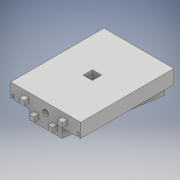
# Autodesk Inventor part: tb3_start
Saved by Autodesk Inventor 2017 (Build 210142000, 142)
## iProperties
Created: 2017-02-24
Part Number: tb3_start
Material: Generic
Document SubType Name: Modeling
Designer: PC
Density: 1 g/cm^3
Appearance: Default
Author: PC
Autodesk Inventor part; units mm, degrees
ref_plane "YZ Plane" through (0, 0, 0) normal (1, 0, 0) x (0, 1, 0)
ref_plane "XZ Plane" through (0, 0, 0) normal (0, 1, 0) x (-1, 0, 0)
ref_plane "XY Plane" through (0, 0, 0) normal (0, 0, 1) x (1, 0, 0)
sketch "Sketch5" plane through (0, 0, 0) normal (0, 1, 0) x (-1, 0, 0)
  line L0 (-37.5, -7.5) -> (37.5, -7.5)
  line L1 (37.5, -7.5) -> (37.5, 7.5)
  line L2 (37.5, 7.5) -> (-37.5, 7.5)
  line L3 (-37.5, 7.5) -> (-37.5, -7.5)
  line L4 (-37.5, -7.5) -> (37.5, 7.5) construction
  line L5 (37.5, -7.5) -> (-37.5, 7.5) construction
  point P0 (0, 0)
  dimension "d6" = 75
  dimension "d7" = 15
  constraints: 12 end point, 2 midpoint, 2 parallel, 1 horizontal, 1 perpendicular
  measures "d6" distance of L2.end L1.end
  measures "d7" distance of L1.end L0.end
extrude "Extrusion2" add sketch "Sketch5" along normal blind 100
sketch "Sketch36" plane through (0, 0, 0) normal (0, -1, 0) x (1, 0, 0)
  line L0 (-37.5, 7.5) -> (37.5, 7.5) projected
  line L1 (0, 7.5) -> (0, -2.5)
  point P0 (0, 0)
  dimension "d82" = 10
  constraints: 2 end point, 1 midpoint, 1 vertical
  measures "d82" distance of L1.start L1.end
hole "Hole1" at (0, 0, -2.5) direction (0, 1, 0) diameter 6.4 depth 10 tip angle 118
sketch "Sketch37" plane through (37.5, 0, -7.5) normal (0, 0, -1) x (-1, 0, 0)
  line L0 (37.5, 0) -> (55, 0)
  line L1 (75, 0) -> (0, 0) projected
  line L2 (70, 0) -> (70, 95)
  line L3 (0, 100) -> (75, 100) projected
  line L4 (70, 0) -> (165, 0) construction
  line L5 (70, 95) -> (5, 95)
  line L6 (0, 0) -> (0, 100) projected
  line L7 (5, 95) -> (5, 0)
  line L8 (5, 0) -> (0, 0)
  line L9 (0, 100) -> (75, 100)
  line L10 (75, 100) -> (75, 0)
  line L11 (55, 0) -> (70, 95)
  line L12 (5, 95) -> (70, 95)
  line L13 (37.5, 0) -> (20, 0)
  line L14 (20, 0) -> (5, 95)
  dimension "d90" = 17.5
  dimension "d91" = 95
  dimension "d92" = 90
  dimension "d93" = 65
  dimension "d94" = 17.5
  constraints: 24 end point, 6 perpendicular, 4 point on line, 2 horizontal, 1 collinear
  measures "d90" distance of L0.start L0.end
  measures "d91" distance of L2.start L2.end
  measures "d92" angle of L4 L2
  measures "d93" distance of L2.end L5.end
  measures "d94" distance of L0.start L13.end
extrude "Extrusion11" add sketch "Sketch37" along normal blind 10 contours L1 L14 L5 L11 L0
sketch "Sketch38" plane through (37.5, 100, -7.5) normal (0, 0, -1) x (-1, 0, 0)
  line L0 (75, -100) -> (0, -100) projected
  line L1 (1.5, -100) -> (3.5, -100)
  line L2 (3.5, -100) -> (3.5, -1.5)
  line L3 (3.5, -1.5) -> (1.5, -1.5)
  line L4 (1.5, -1.5) -> (1.5, -100)
  line L5 (1.5, -1.5) -> (73.5, -1.5)
  line L6 (73.5, -1.5) -> (73.5, -3)
  line L7 (73.5, -3) -> (1.5, -3)
  line L8 (1.5, -3) -> (1.5, -1.5)
  line L9 (55, -100) -> (75, -100) projected
  line L10 (73.5, -1.5) -> (71.5, -1.5)
  line L11 (71.5, -1.5) -> (71.5, -100)
  line L12 (71.5, -100) -> (73.5, -100)
  line L13 (73.5, -100) -> (73.5, -1.5)
  point P0 (37.5, -100)
  dimension "d97" = 2
  dimension "d98" = 98.5
  dimension "d99" = 72
  dimension "d100" = 2
  constraints: 24 end point, 6 parallel, 3 horizontal, 3 perpendicular, 2 point on line
  measures "d97" distance of L3.end L2.end
  measures "d98" distance of L2.end L1.end
  measures "d99" distance of L6.end L7.end
  measures "d100" distance of L12.end L11.end
extrude "Extrusion12" cut sketch "Sketch38" against normal blind 5 contours L0 L11 L7 L13 | L7 L11 L5 L6 | L7 L2 L5 L11 | L0 L4 L7 L2 | L7 L4 L3 L2
sketch "Sketch39" plane through (-37.5, 0, 7.5) normal (0, 0, 1) x (1, 0, 0)
  line L0 (42.5, 55) -> (32.5, 55)
  line L1 (32.5, 55) -> (32.5, 45)
  line L2 (32.5, 45) -> (42.5, 45)
  line L3 (42.5, 45) -> (42.5, 55)
  line L4 (42.5, 55) -> (32.5, 45) construction
  line L5 (32.5, 55) -> (42.5, 45) construction
  point P0 (37.5, 0)
  point P1 (37.5, 50)
  dimension "d103" = 10
  dimension "d104" = 10
  constraints: 12 end point, 2 midpoint, 2 parallel, 1 horizontal, 1 perpendicular
  measures "d103" distance of L2.end L1.end
  measures "d104" distance of L1.end L0.end
extrude "Extrusion13" cut sketch "Sketch39" against normal blind 10
sketch "Sketch43" plane through (0, 0, 0) normal (0, -1, 0) x (1, 0, 0)
  line L0 (17.5, -7.5) -> (17.5, -17.5) projected
  line L1 (17.5, -17.5) -> (12.5, -17.5)
  line L2 (12.5, -17.5) -> (12.5, -12.5)
  line L3 (12.5, -12.5) -> (17.5, -12.5)
  line L4 (17.5, -12.5) -> (17.5, -17.5)
  line L5 (12.5, -12.5) -> (7.5, -12.5)
  line L6 (7.5, -12.5) -> (7.5, -7.5)
  line L7 (7.5, -7.5) -> (12.5, -7.5)
  line L8 (12.5, -7.5) -> (12.5, -12.5)
  point P0 (0, 0)
  dimension "d122" = 5
  dimension "d123" = 5
  dimension "d124" = 5
  dimension "d125" = 5
  constraints: 16 end point, 4 parallel, 2 horizontal, 2 perpendicular
  measures "d122" distance of L2.end L3.end
  measures "d123" distance of L1.end L2.end
  measures "d124" distance of L6.end L7.end
  measures "d125" distance of L5.end L6.end
extrude "Extrusion16" add sketch "Sketch43" along normal blind 5 contours L5 L6 L7 L8
sketch "Sketch45" plane through (0, 0, 0) normal (0, -1, 0) x (1, 0, 0)
  line L0 (-17.5, -7.5) -> (-17.5, -17.5) projected
  line L1 (-17.5, -17.5) -> (-12.5, -17.5)
  line L2 (-12.5, -17.5) -> (-12.5, -12.5)
  line L3 (-12.5, -12.5) -> (-17.5, -12.5)
  line L4 (-17.5, -12.5) -> (-17.5, -17.5)
  line L5 (-12.5, -12.5) -> (-7.5, -12.5)
  line L6 (-7.5, -12.5) -> (-7.5, -7.5)
  line L7 (-7.5, -7.5) -> (-12.5, -7.5)
  line L8 (-12.5, -7.5) -> (-12.5, -12.5)
  point P0 (0, 0)
  dimension "d128" = 5
  dimension "d129" = 5
  dimension "d130" = 5
  dimension "d131" = 5
  constraints: 16 end point, 4 parallel, 2 horizontal, 2 perpendicular
  measures "d128" distance of L3.end L2.end
  measures "d129" distance of L2.end L1.end
  measures "d130" distance of L7.end L6.end
  measures "d131" distance of L6.end L5.end
extrude "Extrusion17" add sketch "Sketch45" along normal blind 5 contours L8 L7 L6 L5
sketch "Sketch48" plane through (0, 0, 0) normal (0, -1, 0) x (1, 0, 0)
  line L0 (-27.5, 7.5) -> (27.5, 7.5)
  line L1 (27.5, 7.5) -> (27.5, -7.5)
  line L2 (27.5, -7.5) -> (-27.5, -7.5)
  line L3 (-27.5, -7.5) -> (-27.5, 7.5)
  line L4 (-27.5, 7.5) -> (27.5, -7.5) construction
  line L5 (27.5, 7.5) -> (-27.5, -7.5) construction
  line L6 (0, -7.5) -> (27.5, -7.5)
  line L7 (27.5, -7.5) -> (27.5, 7.5)
  line L8 (27.5, 7.5) -> (0, 7.5)
  line L9 (0, 7.5) -> (0, -7.5)
  line L10 (13.75, -7.5) -> (27.5, -7.5)
  line L11 (27.5, -7.5) -> (27.5, 7.5)
  line L12 (27.5, 7.5) -> (13.75, 7.5)
  line L13 (13.75, 7.5) -> (13.75, -7.5)
  line L14 (20.625, -7.5) -> (27.5, -7.5)
  line L15 (27.5, -7.5) -> (27.5, 7.5)
  line L16 (27.5, 7.5) -> (20.625, 7.5)
  line L17 (20.625, 7.5) -> (20.625, -7.5)
  line L18 (18.125, 2.5) -> (23.125, 2.5)
  line L19 (23.125, 2.5) -> (23.125, -2.5)
  line L20 (23.125, -2.5) -> (18.125, -2.5)
  line L21 (18.125, -2.5) -> (18.125, 2.5)
  line L22 (18.125, 2.5) -> (23.125, -2.5) construction
  line L23 (23.125, 2.5) -> (18.125, -2.5) construction
  point P0 (0, 0)
  point P1 (20.625, 0)
  dimension "d145" = 55
  dimension "d146" = 15
  dimension "d147" = 5
  dimension "d148" = 5
  constraints: 48 end point, 10 parallel, 8 midpoint, 5 horizontal, 5 perpendicular
  measures "d145" distance of L1.end L2.end
  measures "d146" distance of L0.end L1.end
  measures "d147" distance of L19.end L20.end
  measures "d148" distance of L18.end L19.end
extrude "Extrusion20" add sketch "Sketch48" along normal blind 5 contours L18 L19 L20 L17 | L17 L20 L21 L18
sketch "Sketch49" plane through (0, 0, 0) normal (0, -1, 0) x (1, 0, 0)
  line L0 (-27.5, 7.5) -> (27.5, 7.5)
  line L1 (27.5, 7.5) -> (27.5, -7.5)
  line L2 (27.5, -7.5) -> (-27.5, -7.5)
  line L3 (-27.5, -7.5) -> (-27.5, 7.5)
  line L4 (-27.5, 7.5) -> (27.5, -7.5) construction
  line L5 (27.5, 7.5) -> (-27.5, -7.5) construction
  line L6 (0, -7.5) -> (-27.5, -7.5)
  line L7 (-27.5, -7.5) -> (-27.5, 7.5)
  line L8 (-27.5, 7.5) -> (0, 7.5)
  line L9 (0, 7.5) -> (0, -7.5)
  line L10 (0, -7.5) -> (-27.5, -7.5)
  line L11 (-27.5, -7.5) -> (-27.5, 7.5)
  line L12 (-27.5, 7.5) -> (0, 7.5)
  line L13 (0, 7.5) -> (0, -7.5)
  line L14 (-13.75, -7.5) -> (-27.5, -7.5)
  line L15 (-27.5, -7.5) -> (-27.5, 7.5)
  line L16 (-27.5, 7.5) -> (-13.75, 7.5)
  line L17 (-13.75, 7.5) -> (-13.75, -7.5)
  line L18 (-20.625, -7.5) -> (-27.5, -7.5)
  line L19 (-27.5, -7.5) -> (-27.5, 7.5)
  line L20 (-27.5, 7.5) -> (-20.625, 7.5)
  line L21 (-20.625, 7.5) -> (-20.625, -7.5)
  line L22 (-23.125, 2.5) -> (-18.125, 2.5)
  line L23 (-18.125, 2.5) -> (-18.125, -2.5)
  line L24 (-18.125, -2.5) -> (-23.125, -2.5)
  line L25 (-23.125, -2.5) -> (-23.125, 2.5)
  line L26 (-23.125, 2.5) -> (-18.125, -2.5) construction
  line L27 (-18.125, 2.5) -> (-23.125, -2.5) construction
  point P0 (0, 0)
  point P1 (-20.625, 0)
  dimension "d151" = 55
  dimension "d152" = 15
  dimension "d153" = 5
  dimension "d154" = 5
  constraints: 56 end point, 12 parallel, 8 midpoint, 6 horizontal, 6 perpendicular
  measures "d151" distance of L1.end L2.end
  measures "d152" distance of L0.end L1.end
  measures "d153" distance of L23.end L24.end
  measures "d154" distance of L22.end L23.end
extrude "Extrusion21" add sketch "Sketch49" along normal blind 5 contours L22 L23 L24 L21 | L21 L24 L25 L22
body "Solid2"
